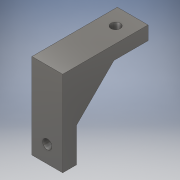
# Autodesk Inventor part: 90degree Braces
Saved by Autodesk Inventor 2019.4 (Build 234330000, 330)
## iProperties
Created: 2019-11-07
Part Number: 90degree Braces
Material: Steel, Cast
Document SubType Name: Modeling
Designer: admin
Density: 7.85 g/cm^3
Appearance: Semi-Polished
Author: admin
Autodesk Inventor part; units mm, degrees
ref_plane "YZ Plane" through (0, 0, 0) normal (1, 0, 0) x (0, 1, 0)
ref_plane "XZ Plane" through (0, 0, 0) normal (0, 1, 0) x (-1, 0, 0)
ref_plane "XY Plane" through (0, 0, 0) normal (0, 0, 1) x (1, 0, 0)
sketch "Sketch1" plane through (0, 0, 0) normal (1, 0, 0) x (0, 1, 0)
  line L0 (-50, 0) -> (0, 0)
  line L1 (0, 0) -> (0, -50)
  line L2 (0, -50) -> (-8, -50)
  line L3 (-8, -50) -> (-8, -30)
  line L4 (-8, -30) -> (-30, -8)
  line L5 (-30, -8) -> (-50, -8)
  line L6 (-50, -8) -> (-50, 0)
  dimension "d0" = 50
  dimension "d1" = 8
  dimension "d2" = 8
  dimension "d3" = 20
  dimension "d4" = 20
  constraints: 14 end point, 4 perpendicular, 2 horizontal, 1 parallel
  measures "d0" distance of L0.end L1.end
  measures "d1" distance of L1.end L2.end
  measures "d2" distance of L5.end L0.start
  measures "d3" distance of L4.end L5.end
  measures "d4" distance of L2.end L3.end
extrude "Extrusion1" add sketch "Sketch1" along normal blind 18
sketch "Sketch2" plane through (0, -8, -50) normal (0, -1, 0) x (1, 0, 0)
  circle A0 centre (9, 10) radius 2.75
  line L0 (18, 20) -> (18, 0) projected
  line L1 (0, 0) -> (18, 0) projected
  point P0 (0, 50)
  dimension "d7" = 5.5
  dimension "d8" = 9
  dimension "d9" = 10
  constraints: 1 centre point
  measures "d7" diameter of A0
  measures "d8" distance from line of L0 A0.centre
  measures "d9" distance from line of L1 A0.centre
extrude "Extrusion2" cut sketch "Sketch2" against normal through all
sketch "Sketch3" plane through (0, -50, -8) normal (0, 0, -1) x (-1, 0, 0)
  circle A0 centre (-9, 10) radius 2.75
  line L0 (-18, 0) -> (-18, 20) projected
  line L1 (0, 0) -> (-18, 0) projected
  point P0 (0, 50)
  dimension "d12" = 5.5
  dimension "d13" = 9
  dimension "d14" = 10
  constraints: 1 centre point
  measures "d12" diameter of A0
  measures "d13" distance from line of L0 A0.centre
  measures "d14" distance from line of L1 A0.centre
extrude "Extrusion3" cut sketch "Sketch3" against normal through all
body "Solid1"
